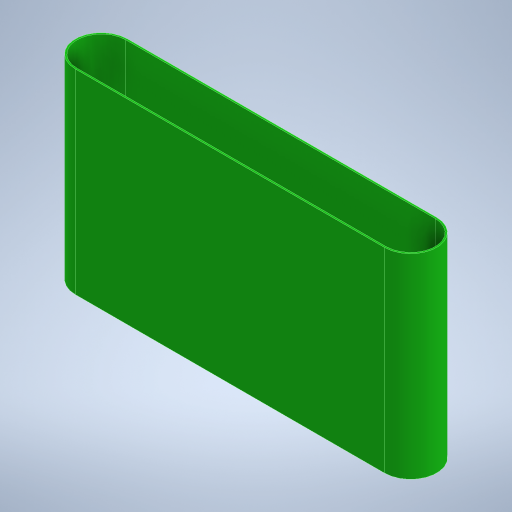
# Autodesk Inventor part: HCMUTE-CDT23-BELT_PHAN_LOAI
Saved by Autodesk Inventor 2023 (Build 270158000, 158)
## iProperties
Created: 2023-10-09
Part Number: HCMUTE-CDT23-BELT_PHAN_LOAI
Material: PVC, Unplasticized
Document SubType Name: Modeling
Designer: havie
Density: 1.29 g/cm^3
Appearance: Dark Green
Author: havie
Autodesk Inventor part; units mm, degrees
ref_plane "YZ Plane" through (0, 0, 0) normal (1, 0, 0) x (0, 1, 0)
ref_plane "XZ Plane" through (0, 0, 0) normal (0, 1, 0) x (-1, 0, 0)
sketch "Sketch1" plane through (0, 0, 0) normal (0, 1, 0) x (-1, 0, 0)
  line L0 (-220, 0) -> (220, 0) construction
  line L1 (-190, -30) -> (190, -30)
  line L2 (190, 30) -> (-190, 30)
  arc A0 (-190, 30) -> (-190, -30) centre (-190, 0) ccw
  arc A1 (190, -30) -> (190, 30) centre (190, 0) ccw
  point P0 (0, 0)
  point P1 (0, 0)
  dimension "d0" = 380
  dimension "d1" = 60
  constraints: 8 end point, 6 point on circle, 4 tangent, 2 centre point, 2 point on line, 1 coincident, 1 horizontal, 1 midpoint, 1 parallel
  measures "d0" distance of A1.centre A0.centre
  measures "d1" distance between parallel lines of L2 L1
ref_plane "Work Plane1" through (220, 0, 0) normal (0, 0, -1) x (-1, 0, 0)
sketch "Sketch2" plane through (220, 0, 0) normal (0, 0, -1) x (-1, 0, 0)
  line L0 (0, 120) -> (-2, 120)
  line L1 (-2, 120) -> (-2, -120)
  line L2 (-2, -120) -> (0, -120)
  line L3 (0, -120) -> (0, 120)
  line L4 (0, 120) -> (-2, -120) construction
  line L5 (-2, 120) -> (0, -120) construction
  point P0 (220, 0)
  point P1 (-1, 0)
  point P2 (-1, -120)
  point P3 (-1, 120)
  point P4 (0, 0)
  point P5 (-2, 0)
  point P6 (0, 0)
  dimension "d2" = 240
  dimension "d3" = 2
  constraints: 12 end point, 6 midpoint, 2 parallel, 1 coincident, 1 horizontal, 1 perpendicular
  measures "d2" distance of point (-1, -120) point (-1, 120)
  measures "d3" distance between parallel lines of L1 L3
sweep "Sweep1" add profiles "Sketch2" path "Sketch1"
body "Solid1"
